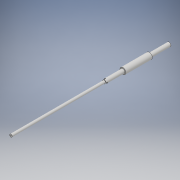
# Autodesk Inventor part: Achse
Saved by Autodesk Inventor 2017 (Build 210142000, 142)
## iProperties
Created: 2019-06-21
Part Number: Achse
Material: Generic
Document SubType Name: Modeling
Designer: Ole Simmering
Density: 1 g/cm^3
Appearance: Default
Author: Ole Simmering
Autodesk Inventor part; units mm, degrees
ref_plane "YZ Plane" through (0, 0, 0) normal (1, 0, 0) x (0, 1, 0)
ref_plane "XZ Plane" through (0, 0, 0) normal (0, 1, 0) x (-1, 0, 0)
ref_plane "XY Plane" through (0, 0, 0) normal (0, 0, 1) x (1, 0, 0)
sketch "Sketch1" plane through (0, 0, 0) normal (0, 0, 1) x (1, 0, 0)
  line L0 (0, 0) -> (0, -500) construction
  line L1 (0, 0) -> (6, 0)
  line L2 (6, 0) -> (6, -60)
  line L3 (6, -60) -> (9.2, -60)
  line L4 (9.2, -60) -> (9.2, -140)
  line L5 (9.2, -140) -> (6, -140)
  line L6 (6, -140) -> (6, -192)
  line L7 (0, 0) -> (0, -480)
  line L8 (0, 0) -> (0, 9) construction
  line L9 (4, -480) -> (4, -192)
  line L10 (4, -192) -> (6, -192)
  line L11 (4, -480) -> (0, -480)
  dimension "d1" = 12
  dimension "d2" = 60
  dimension "d3" = 18.4
  dimension "d4" = 80
  dimension "d7" = 8
  dimension "d8" = 288
  dimension "d9" = 480
  constraints: 24 end point, 5 perpendicular, 4 vertical, 2 collinear, 2 horizontal, 1 point on line
  measures "d1" diameter of L2 L0
  measures "d2" distance of L1.end L2.end
  measures "d3" diameter of L4 L0
  measures "d4" distance of L3.end L4.end
  measures "d7" diameter of L9 L0
  measures "d8" distance of L9.start L9.end
  measures "d9" distance between parallel lines of L1 L11
revolve "Revolution1" add sketch "Sketch1" angle 360 about axis through (0, 0, 0) along (0, -1, 0)
sketch "Sketch2" plane through (0, -192, 0) normal (0, -1, 0) x (1, 0, 0)
  line L0 (0, 0) -> (0, 10.7217) construction
  line L1 (0, 0) -> (0, -10) construction
  line L2 (0, 0) -> (-12.4689, 0) construction
  line L3 (0, 0) -> (11.6918, 0) construction
  circle A0 centre (0, 0) radius 6 construction
  arc A1 (6, 0) -> (0, 6) centre (0, 0) ccw
  arc A2 (-6, 0) -> (0, -6) centre (0, 0) ccw
  arc A3 (4, 0) -> (0, 4) centre (0, 0) ccw
  arc A4 (-4, 0) -> (0, -4) centre (0, 0) ccw
  line L4 (-4, 0) -> (-6, 0)
  line L5 (0, -4) -> (0, -6)
  line L6 (0, 4) -> (0, 6)
  line L7 (4, 0) -> (6, 0)
  dimension "d10" = 4
  dimension "d11" = 4
  constraints: 16 end point, 10 point on circle, 6 point on line, 4 centre point, 4 coincident, 3 collinear, 2 vertical, 1 horizontal, 1 perpendicular
  measures "d10" radius of A3
  measures "d11" radius of A4
extrude "Extrusion1" add sketch "Sketch2" along normal blind 5
sketch "Sketch3" plane through (0, -480, 0) normal (0, -1, 0) x (1, 0, 0)
  point P0 (0, 0)
  point P1 (0, 0)
  constraints: 1 coincident
hole "Hole1" at (0, -480, 0) direction (0, 1, 0) diameter 1.567 depth 6.3 tip angle 118 thread size "M2x0.4" class "6H" standard "ANSI Metric M Profile"
sketch "Sketch4" plane through (0, -480, 0) normal (0, -1, 0) x (1, 0, 0)
  point P0 (0, 0)
hole "Hole2" at (0, -480, 0) direction (0, 1, 0) diameter 1.567 depth 5 tip angle 120 thread size "M2x0.4" class "6H" standard "ISO Metric profile"
body "Solid1"
